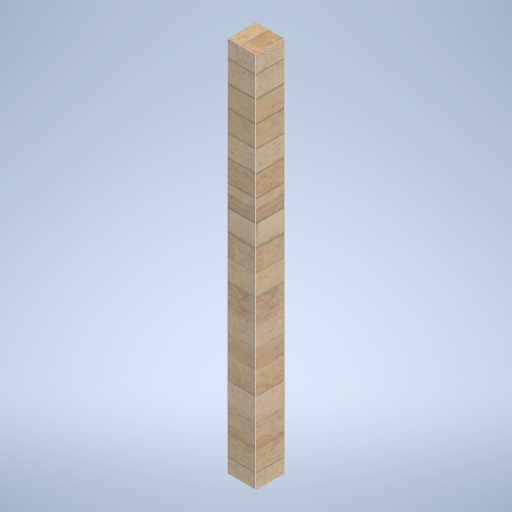
# Autodesk Inventor part: Soporte
Saved by Autodesk Inventor 2025.3 (Build 293356000, 356)
## iProperties
Created: 2025-11-02
Part Number: Soporte
Material: Madera (arce)
Document SubType Name: Modeling
Designer: PAVILION
Density: 0.67 g/cm^3
Appearance: Arce natural - De color oscuro brillante
Author: PAVILION
Autodesk Inventor part; units mm, degrees
ref_plane "YZ Plane" through (0, 0, 0) normal (1, 0, 0) x (0, 1, 0)
ref_plane "XZ Plane" through (0, 0, 0) normal (0, 1, 0) x (-1, 0, 0)
ref_plane "XY Plane" through (0, 0, 0) normal (0, 0, 1) x (1, 0, 0)
sketch "Boceto1" plane through (0, 0, 0) normal (0, 1, 0) x (-1, 0, 0)
  line L0 (37.5, 37.5) -> (-37.5, 37.5)
  line L1 (-37.5, 37.5) -> (-37.5, -37.5)
  line L2 (-37.5, -37.5) -> (37.5, -37.5)
  line L3 (37.5, -37.5) -> (37.5, 37.5)
  line L4 (37.5, 37.5) -> (-37.5, -37.5) construction
  line L5 (-37.5, 37.5) -> (37.5, -37.5) construction
  point P0 (0, 0)
  dimension "d0" = 75
  dimension "d1" = 75
  constraints: 12 end point, 2 midpoint, 2 parallel, 1 horizontal, 1 perpendicular
  measures "d0" distance of L2.end L0.start
  measures "d1" distance of L1.end L2.end
extrude "Extrusión1" add sketch "Boceto1" along normal mid plane 1000
